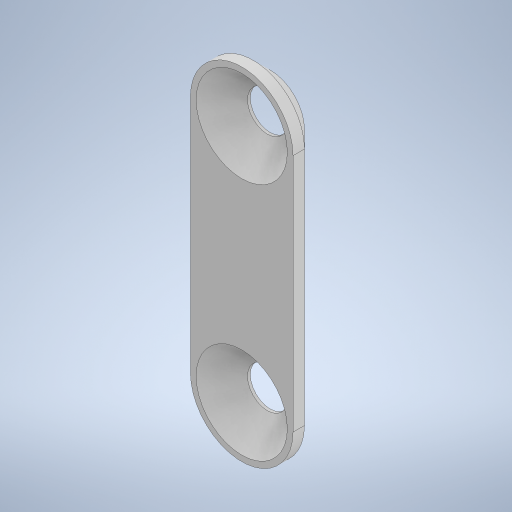
# Autodesk Inventor part: zaslepka
Saved by Autodesk Inventor 2023 (Build 270158000, 158)
## iProperties
Created: 2023-08-18
Part Number: zaslepka
Material: Ogólny
Document SubType Name: Modeling
Designer: Kamil
Density: 1 g/cm^3
Appearance: Domyślna
Author: Kamil
Autodesk Inventor part; units mm, degrees
ref_plane "YZ Plane" through (0, 0, 0) normal (1, 0, 0) x (0, 1, 0)
ref_plane "XZ Plane" through (0, 0, 0) normal (0, 1, 0) x (-1, 0, 0)
sketch "Szkic1" plane through (0, 0, 0) normal (0, 0, 1) x (1, 0, 0)
  line L0 (-17.5, 39.3937) -> (-17.5, -45.2473) projected
  line L1 (17.5, -26.5287) -> (-17.5, -45.2473) projected
  line L2 (17.5, 40.0799) -> (17.5, -26.5287) projected
  arc A0 (17.5, 40.0799) -> (16.7161, 41.0563) centre (16.5, 40.0799) ccw projected
  line L3 (3.9006, 43.8921) -> (16.7161, 41.0563) projected
  arc A1 (3.9006, 43.8921) -> (3.7868, 43.9105) centre (3.6845, 42.9157) ccw projected
  line L4 (3.7868, 43.9105) -> (-8.4909, 46.6272) projected
  arc A2 (-8.4909, 46.6272) -> (-17.5, 39.3937) centre (-10.0915, 39.3937) ccw projected
  line L5 (8.675, 4.2897) -> (8.675, -16.7103) projected
  arc A3 (-1.325, -16.7103) -> (8.675, -16.7103) centre (3.675, -16.7103) ccw projected
  line L6 (-1.325, -16.7103) -> (-1.325, 4.2897) projected
  arc A4 (8.675, 4.2897) -> (-1.325, 4.2897) centre (3.675, 4.2897) ccw projected
  point P0 (0, 0)
ref_plane "Płaszczyzna konstrukcyjna1" through (-1.325, -21.7103, -2.5) normal (0, 0, 1) x (1, 0, 0)
extrude "Wyciągnięcie proste1" add sketch "Szkic1" against normal up to surface (2.5 mm away) contours L5 A3 L6 A4
sketch "Szkic2" plane through (0, 0, 0) normal (0, 0, 1) x (1, 0, 0)
  circle A0 centre (3.675, 4.2897) radius 1.5 projected
  circle A1 centre (3.675, -16.7103) radius 1.5 projected
  arc A2 (8.675, 4.2897) -> (-1.325, 4.2897) centre (3.675, 4.2897) ccw projected
  point P0 (0, 0)
  constraints: 2 coincident
hole "Otwór1" at (3.675, 4.2897, 0) at (3.675, -16.7103, 0) direction (0, 0, -1) diameter 3.5 end through all countersink diameter 8 countersink angle 90
sketch "Szkic3" plane through (0, 0, 0) normal (0, 0, 1) x (1, 0, 0)
  circle A0 centre (3.675, 4.2897) radius 1.75 projected
  circle A1 centre (3.675, -16.7103) radius 1.75 projected
  circle A2 centre (3.675, 4.2897) radius 4 projected
  circle A3 centre (3.675, -16.7103) radius 4 projected
  line L0 (8.675, -16.7103) -> (8.675, 4.2897) projected
  arc A4 (8.675, 4.2897) -> (-1.325, 4.2897) centre (3.675, 4.2897) ccw projected
  line L1 (-1.325, 4.2897) -> (-1.325, -16.7103) projected
  arc A5 (-1.325, -16.7103) -> (8.675, -16.7103) centre (3.675, -16.7103) ccw projected
  arc A6 (8.175, 4.2897) -> (-0.825, 4.2897) centre (3.675, 4.2897) ccw
  line L2 (8.175, 4.2897) -> (8.175, -16.7103)
  arc A7 (-0.825, -16.7103) -> (8.175, -16.7103) centre (3.675, -16.7103) ccw
  line L3 (-0.825, -16.7103) -> (-0.825, 4.2897)
  point P0 (0, 0)
  dimension "d9" = 0.5
  constraints: 4 end point, 4 point on circle, 2 centre point, 3 other
  measures "d9" radial gap between concentric circles of A4 A6
extrude "Wyciągnięcie proste2" cut sketch "Szkic3" against normal through all contours A5 L1 A4 L0
chamfer "Faza1" distance 1.5 angle 45 4 edges at (3.675, -21.2103, -2.5) (-0.825, -6.2103, -2.5) (3.675, 8.7897, -2.5) (8.175, -6.2103, -2.5)
